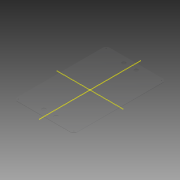
# Autodesk Inventor part: D-051
Saved by Autodesk Inventor 2015 (Build 190159000, 159)
## iProperties
Company: MARCHA TECHNOLOGY
Created: 2013-10-01
Part Number: D-051
Document SubType Name: Modeling
Designer: O.Martin
Density: 1.06 g/cm^3
Project: WITBOXprinter_K01
Material: ABS Plastic
Description: TAPA SUPERIOR
Stock Number: 28655
Mass: 190.66 g
Surface Area: 1827.51 cm^2
Volume: 179.868 cm^3
Appearance: Clear - Light
Author: O.Martin
Autodesk Inventor part; units mm, degrees
ref_plane "XY Plane" through (0, 0, 0) normal (0, 0, 1) x (1, 0, 0)
sketch "Boceto1" plane through (0, 0, 0) normal (0, 0, 1) x (1, 0, 0)
  line L0 (-121.5, -187) -> (121.5, -187)
  line L1 (121.5, -187) -> (121.5, 187)
  line L2 (121.5, 187) -> (-121.5, 187)
  line L3 (-121.5, 187) -> (-121.5, -187)
  line L4 (111.5, 187) -> (121.5, 177)
  line L5 (121.5, -177) -> (111.5, -187)
  line L6 (-111.5, -187) -> (-121.5, -177)
  line L7 (-111.5, 187) -> (-121.5, 177)
  point P0 (0, 0)
  point P1 (0, -187)
  point P2 (121.5, 0)
  dimension "d0" = 243
  dimension "d1" = 374
  dimension "d8" = 45
  dimension "d9" = 10
  constraints: 16 end point, 8 point on line, 7 perpendicular, 2 midpoint, 2 parallel, 1 horizontal, 1 horizontal alignment, 1 vertical alignment
  measures "d0" distance of L1.end L2.end
  measures "d1" distance of L0.end L1.end
  measures "d8" angle of L2 L4
  measures "d9" distance from line of L4.end L2
extrude "Extrusión1" add sketch "Boceto1" along normal blind 2 contours L6 L3 L7 L2 L4 L1 L5 L0
fillet "Empalme2" radius 4 8 edges at (121.5, 177, 1) (111.5, 187, 1) (-111.5, 187, 1) (-121.5, 177, 1) (-121.5, -177, 1) (-111.5, -187, 1) (121.5, -177, 1) (111.5, -187, 1)
sketch "Boceto2" plane through (0, 0, 2) normal (0, 0, 1) x (1, 0, 0)
  line L0 (-121.5, -175.3431) -> (-121.5, 175.3431) projected
  line L1 (-109.8431, 187) -> (109.8431, 187) projected
  line L2 (-112, 177.5) -> (112, 177.5) construction
  line L3 (112, 177.5) -> (112, -177.5) construction
  line L4 (112, -177.5) -> (-112, -177.5) construction
  line L5 (-112, -177.5) -> (-112, 177.5) construction
  point P0 (-112, 0)
  point P1 (-121.5, 0)
  point P2 (0, 187)
  point P3 (0, 177.5)
  dimension "d11" = 224
  dimension "d12" = 355
  constraints: 8 end point, 4 coincident, 4 midpoint, 2 parallel, 1 horizontal, 1 horizontal alignment, 1 perpendicular, 1 vertical alignment
  measures "d11" distance of L3.end L4.end
  measures "d12" distance of L2.end L3.end
hole "Agujero1" at (112, 177.5, 2) at (-112, 177.5, 2) at (-112, -177.5, 2) at (112, -177.5, 2) direction (0, 0, -1) diameter 3.5 depth 8 tip angle 118
sketch "Boceto3" plane through (0, 0, 2) normal (0, 0, 1) x (1, 0, 0)
  line L0 (-121.5, -175.3431) -> (-121.5, 175.3431) projected
  line L1 (-109.8431, 187) -> (109.8431, 187) projected
  line L2 (-25, 162) -> (25, 162) construction
  line L3 (25, 162) -> (25, -162) construction
  line L4 (25, -162) -> (-25, -162) construction
  line L5 (-25, -162) -> (-25, 162) construction
  circle A0 centre (-25, 162) radius 7.5
  circle A1 centre (25, 162) radius 7.5
  circle A2 centre (-25, -162) radius 7.5
  circle A3 centre (25, -162) radius 7.5
  point P0 (0, 162)
  point P1 (0, 187)
  point P2 (-25, 0)
  point P3 (-121.5, 0)
  dimension "d20" = 50
  dimension "d21" = 25
  dimension "d22" = 15
  dimension "d23" = 15
  constraints: 8 end point, 4 centre point, 4 coincident, 4 midpoint, 2 equal radius, 2 parallel, 1 horizontal, 1 horizontal alignment, 1 perpendicular, 1 vertical alignment
  measures "d20" distance of L2.start L2.end
  measures "d21" distance between parallel lines of L1 L2
  measures "d22" diameter of A2
  measures "d23" diameter of A3
extrude "Extrusión2" cut sketch "Boceto3" against normal blind 10
body "Solid1"
